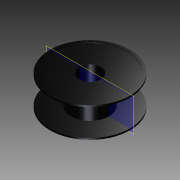
# Autodesk Inventor part: SpoolFilamentToyBuilder
Saved by Autodesk Inventor 2015 SP1 (Build 190203100, 203)
## iProperties
Created: 2014-05-26
Part Number: SpoolFilamentToyBuilder
Material: ABS Plastic
Document SubType Name: Modeling
Designer: Jack
Density: 1.06 g/cm^3
Appearance: Smooth - Black
Mass: 561.038 g
Surface Area: 1478.17 cm^2
Volume: 529.281 cm^3
Author: Jack
Title: Filament Spool
Autodesk Inventor part; units mm, degrees
ref_plane "YZ Plane" through (0, 0, 0) normal (1, 0, 0) x (0, 1, 0)
ref_plane "XZ Plane" through (0, 0, 0) normal (0, 1, 0) x (-1, 0, 0)
ref_plane "XY Plane" through (0, 0, 0) normal (0, 0, 1) x (1, 0, 0)
sketch "Sketch11" plane through (0, 0, 0) normal (0, 0, 1) x (1, 0, 0)
  circle A0 centre (0, 0) radius 100
  dimension "d39" = 200
  constraints: 1 centre point, 1 coincident
  measures "d39" diameter of A0
extrude "Extrusion10" add sketch "Sketch11" along normal blind 4
sketch "Sketch12" plane through (0, 0, 4) normal (0, 0, 1) x (1, 0, 0)
  circle A0 centre (0, 0) radius 100 projected
  circle A1 centre (0, 0) radius 92.5
  dimension "d42" = 185
  constraints: 1 centre point, 1 coincident
  measures "d42" diameter of A1
extrude "Extrusion11" cut sketch "Sketch12" against normal blind 1 contours A1
ref_plane "Work Plane1" through (0, 0, -33.5) normal (0, 0, -1) x (-1, 0, 0)
mirror "Mirror1" about plane through (0, 0, -33.5) normal (0, 0, -1)
sketch "Sketch14" plane through (0, 0, -67) normal (0, 0, 1) x (1, 0, 0)
  circle A0 centre (0, 0) radius 100 projected
  circle A1 centre (0, 0) radius 47.5
  dimension "d46" = 95
  constraints: 1 centre point, 1 coincident
  measures "d46" diameter of A1
extrude "Extrusion12" add sketch "Sketch14" along normal up to next contours A1
sketch "Sketch15" plane through (0, 0, -70) normal (0, 0, -1) x (-1, 0, 0)
  circle A0 centre (0, 0) radius 92.5 projected
  circle A1 centre (0, 0) radius 27
  dimension "d50" = 54
  constraints: 1 centre point, 1 coincident
  measures "d50" diameter of A1
extrude "Extrusion13" cut sketch "Sketch15" against normal up to surface (73 mm away) contours A1
body "Solid2"
